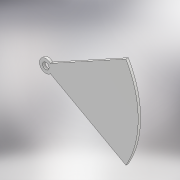
# Autodesk Inventor part: RailBase
Saved by Autodesk Inventor 2018 (Build 220112000, 112)
## iProperties
Created: 2018-03-27
Part Number: RailBase
Material: ABS Plastic
Document SubType Name: Modeling
Designer: mansu
Density: 1.06 g/cm^3
Appearance: Smooth - White
Author: mansu
Autodesk Inventor part; units mm, degrees
ref_plane "YZ Plane" through (0, 0, 0) normal (1, 0, 0) x (0, 1, 0)
ref_plane "XZ Plane" through (0, 0, 0) normal (0, 1, 0) x (-1, 0, 0)
ref_plane "XY Plane" through (0, 0, 0) normal (0, 0, 1) x (1, 0, 0)
sketch "Sketch1" plane through (0, 0, 0) normal (0, 1, 0) x (-1, 0, 0)
  circle A0 centre (0, 0) radius 4
  arc A1 (-86.6006, 50.0033) -> (-86.6006, -50.0033) centre (0, 0) ccw construction
  arc A2 (-90.9833, 52.4122) -> (-90.9833, -52.4122) centre (0, 0) ccw construction
  arc A3 (-5.7479, -5.5643) -> (-5.7479, 5.5643) centre (0, 0) ccw
  line L0 (-5.7479, -5.5643) -> (-100.1431, -57.4467)
  arc A4 (-100.1431, 57.4467) -> (-100.1431, -57.4467) centre (0, 0) ccw
  line L1 (-5.7479, 5.5643) -> (-100.1431, 57.4467)
  point P0 (-115.4502, 0)
  dimension "d0" = 8
  dimension "d1" = 100
  dimension "d2" = 105
  dimension "d3" = 8
  constraints: 9 point on circle, 5 centre point, 4 concentric, 4 end point, 4 point on line, 1 coincident, 1 horizontal alignment, 1 vertical alignment
  measures "d0" diameter of A0
  measures "d1" radius of A1
  measures "d2" radius of A2
  measures "d3" radius of A3
extrude "Extrusion1" add sketch "Sketch1" along normal blind 3
body "Solid1"
